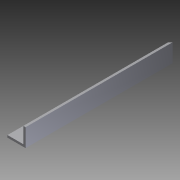
# Autodesk Inventor part: backwards L frame
Saved by Autodesk Inventor 2012 (Build 160160000, 160)
## iProperties
Created: 2012-08-14
Part Number: backwards L frame
Material: Default
Document SubType Name: Modeling
Designer: Bryce
Density: 1 g/cm^3
Author: Bryce
Autodesk Inventor part; units mm, degrees
ref_plane "YZ Plane" through (0, 0, 0) normal (1, 0, 0) x (0, 1, 0)
ref_plane "XZ Plane" through (0, 0, 0) normal (0, 1, 0) x (-1, 0, 0)
ref_plane "XY Plane" through (0, 0, 0) normal (0, 0, 1) x (1, 0, 0)
sketch "Sketch1" plane through (0, 0, 0) normal (0, 0, 1) x (1, 0, 0)
  line L0 (-25.4, 3.175) -> (-3.175, 3.175)
  line L1 (0, 0) -> (-25.4, 0)
  line L2 (-25.4, 0) -> (-25.4, 3.175)
  line L3 (-3.175, 25.4) -> (0, 25.4)
  line L4 (0, 25.4) -> (0, 0)
  line L5 (-3.175, 3.175) -> (-3.175, 25.4)
  dimension "d0" = 25.4
  dimension "d1" = 25.4
  dimension "d2" = 3.175
  dimension "d3" = 3.175
  constraints: 13 end point, 3 perpendicular, 2 parallel, 1 horizontal
  measures "d0" distance of L3.end L1.start
  measures "d1" distance of L1.start L1.end
  measures "d2" distance of L3.start L3.end
  measures "d3" distance of L1.end L0.start
extrude "Extrusion1" add sketch "Sketch1" along normal blind 206.375
sketch "Sketch2" plane through (-25.4, 0, 0) normal (0, -1, 0) x (1, 0, 0)
  line L0 (0, 0) -> (0, 206.375) projected
  line L1 (0, 0) -> (25.4, 0) projected
  line L2 (0, 25.4) -> (25.4, 0)
  dimension "d8" = 45
  constraints: 2 end point, 1 point on line
  measures "d8" angle of L1 L2
extrude "Extrusion2" cut sketch "Sketch2" against normal blind 203.2
sketch "Sketch3" plane through (-25.4, 3.175, 206.375) normal (0, 1, 0) x (1, 0, 0)
  line L0 (0, 0) -> (22.225, 0) projected
  line L1 (22.225, 203.2) -> (22.225, 0) projected
  circle A0 centre (12.7, 114.3) radius 3.175
  point P0 (25.4, 206.375)
  dimension "d11" = 6.35
  dimension "d12" = 114.3
  dimension "d13" = 9.525
  constraints: 1 centre point
  measures "d11" diameter of A0
  measures "d12" distance from line of L0 A0.centre
  measures "d13" distance from line of L1 A0.centre
extrude "Extrusion3" cut sketch "Sketch3" against normal blind 25.4
body "Solid1"
